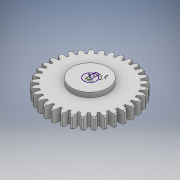
# Autodesk Inventor part: 도면2-3번
Saved by Autodesk Inventor 2018.3 (Build 223284000, 284)
## iProperties
Created: 2019-10-10
Part Number: 도면2-3번
Material: 일반
Document SubType Name: Modeling
Designer: MyTool
Density: 1 g/cm^3
Appearance: 기본값
Author: MyTool
Autodesk Inventor part; units mm, degrees
ref_plane "YZ Plane" through (0, 0, 0) normal (1, 0, 0) x (0, 1, 0)
ref_plane "XZ Plane" through (0, 0, 0) normal (0, 1, 0) x (-1, 0, 0)
ref_plane "XY Plane" through (0, 0, 0) normal (0, 0, 1) x (1, 0, 0)
sketch "스케치1" plane through (0, 0, 0) normal (0, 0, 1) x (1, 0, 0)
  circle A0 centre (0, 0) radius 33 construction
  circle A1 centre (0, 0) radius 35 construction
  circle A2 centre (0, 0) radius 30 construction
  line L0 (0, 35) -> (0, 0) construction
  line L1 (0.57, 34.9954) -> (0.57, 0) construction
  line L2 (1.57, 32.9626) -> (1.57, 0) construction
  line L3 (2.07, 29.9285) -> (2.07, 0) construction
  arc A3 (2.07, 29.9285) -> (0.5982, 34.9949) centre (-7.386, 29.9285) ccw
  arc A4 (-0.5982, 34.9949) -> (-2.07, 29.9285) centre (7.386, 29.9285) ccw
  arc A5 (-2.07, 29.9285) -> (2.07, 29.9285) centre (0, 0) ccw
  arc A6 (0.5982, 34.9949) -> (-0.5982, 34.9949) centre (0, 0) ccw
  dimension "d0" = 66
  dimension "d2" = 60
  dimension "d1" = 70
  dimension "d4" = 1
  dimension "d5" = 0.5
  dimension "d6" = 1.57
  constraints: 14 point on circle, 8 end point, 5 centre point, 5 coincident, 4 vertical, 3 symmetric about line, 1 tangent, 7 other
  measures "d1" diameter of A1
  measures "d4" distance between parallel lines of L2 L1
  measures "d5" distance between parallel lines of L3 L2
  measures "d6" distance between parallel lines of L2 L0
extrude "돌출1" add sketch "스케치1" along normal mid plane 10
chamfer "모따기1" distance 1 angle 45 2 edges at (0, 35, -5) (0, 35, 5)
pattern_circular "원형 패턴1" count 33 over 360 about axis through (0, 0, 0) along (0, 0, 1) of "돌출1", "모따기1"
sketch "스케치2" plane through (0, 0, 5) normal (0, 0, 1) x (1, 0, 0)
  circle A0 centre (0, 0) radius 15
  dimension "d15" = 30
  constraints: 1 centre point, 1 coincident
  measures "d15" diameter of A0
extrude "돌출2" add sketch "스케치2" along normal blind 4
mirror "미러1" about plane through (0, 0, 0) normal (0, 0, 1) of "돌출2"
sketch "스케치3" plane through (0, 0, 9) normal (0, 0, 1) x (1, 0, 0)
  circle A0 centre (0, 0) radius 5
  line L0 (-1.5, -1.6) -> (1.5, -1.6)
  line L1 (1.5, -1.6) -> (1.5, 6.4)
  line L2 (1.5, 6.4) -> (-1.5, 6.4)
  line L3 (-1.5, 6.4) -> (-1.5, -1.6)
  dimension "d18" = 10
  dimension "d19" = 1.4
  dimension "d20" = 3
  dimension "d21" = 1.5
  constraints: 8 end point, 2 parallel, 1 centre point, 1 coincident, 1 horizontal, 1 perpendicular
  measures "d18" diameter of A0
  measures "d19" distance edge to line of A0 L2
  measures "d20" distance between parallel lines of L1 L3
  measures "d21" distance from line of point (0, 0) L3
